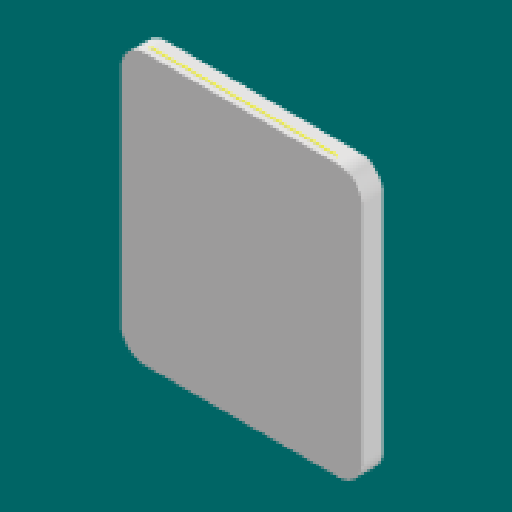
# Autodesk Inventor part: part1
Saved by Autodesk Inventor 2025.2 (Build 292293000, 293)
## iProperties
Created: 2025-05-26
Part Number: part1
Material: Generic
Document SubType Name: Modeling
Designer: ia088
Density: 1 g/cm^3
Appearance: Default
Author: ia088
Autodesk Inventor part; units mm, degrees
ref_plane "YZ Plane" through (0, 0, 0) normal (1, 0, 0) x (0, 1, 0)
ref_plane "XZ Plane" through (0, 0, 0) normal (0, 1, 0) x (-1, 0, 0)
ref_plane "XY Plane" through (0, 0, 0) normal (0, 0, 1) x (1, 0, 0)
ref_plane "Work Plane1" through (0, 0, 0) normal (0, 0, 1) x (1, 0, 0)
sketch "Sketch1" plane through (0, 0, 0) normal (0, 0, 1) x (1, 0, 0)
  line L0 (8.1543, -68.045) -> (8.1793, 2.155) projected
  line L1 (5.1793, 5.155) -> (-55.5957, 5.155) projected
  line L2 (-55.6207, -71.045) -> (5.1543, -71.045) projected
  line L3 (-58.5957, 2.155) -> (-58.6207, -68.045) projected
  arc A0 (8.1793, 2.155) -> (5.1793, 5.155) centre (5.1793, 2.155) ccw projected
  arc A1 (5.1543, -71.045) -> (8.1543, -68.045) centre (5.1543, -68.045) ccw projected
  arc A2 (-58.6207, -68.045) -> (-55.6207, -71.045) centre (-55.6207, -68.045) ccw projected
  arc A3 (-55.5957, 5.155) -> (-58.5957, 2.155) centre (-55.5957, 2.155) ccw projected
  circle A4 centre (-2.54, -13.97) radius 1.7875 projected
  circle A5 centre (-2.54, -13.97) radius 1.5875 projected
  circle A6 centre (-7.62, -66.04) radius 1.7875 projected
  circle A7 centre (-7.62, -66.04) radius 1.5875 projected
  circle A8 centre (-50.8, -15.24) radius 1.7875 projected
  circle A9 centre (-50.8, -15.24) radius 1.5875 projected
  circle A10 centre (-35.56, -66.04) radius 1.7875 projected
  circle A11 centre (-35.56, -66.04) radius 1.5875 projected
  line L4 (9.1793, 2.1536) -> (9.1543, -68.0464)
  arc A12 (5.1543, -72.045) -> (9.1543, -68.0464) centre (5.1543, -68.045) ccw
  line L5 (5.1543, -72.045) -> (-55.6207, -72.045)
  arc A13 (-59.6207, -68.0436) -> (-55.6207, -72.045) centre (-55.6207, -68.045) ccw
  line L6 (-59.6207, -68.0436) -> (-59.5957, 2.1564)
  arc A14 (-55.5957, 6.155) -> (-59.5957, 2.1564) centre (-55.5957, 2.155) ccw
  line L7 (-55.5957, 6.155) -> (5.1793, 6.155)
  arc A15 (9.1793, 2.1536) -> (5.1793, 6.155) centre (5.1793, 2.155) ccw
  point P0 (0, 0)
  dimension "d0" = 1
  constraints: 8 end point, 8 point on circle, 4 centre point, 7 other
  measures "d0" distance between parallel lines of L0 L4
extrude "Extrusion1" add sketch "Sketch1" along normal blind 2 contours A1 L2 A2 L3 A3 L1 A0 L0 | A4 | A5 | A6 | A7 | A8 | A9 | A10 | A11 | L4 A12 L5 A13 L6 A14 L7 A15
sketch "Sketch2" plane through (0, 0, 0) normal (0, 0, -1) x (-1, 0, 0)
  circle A0 centre (35.56, -66.04) radius 1.7875 projected
  circle A1 centre (7.62, -66.04) radius 1.5875 projected
  circle A2 centre (35.56, -66.04) radius 1.5875 projected
  circle A3 centre (50.8, -15.24) radius 1.5875 projected
  circle A4 centre (2.54, -13.97) radius 1.5875 projected
  circle A5 centre (50.8, -15.24) radius 1.4875
  circle A6 centre (2.54, -13.97) radius 1.4875
  circle A7 centre (35.56, -66.04) radius 1.4875
  circle A8 centre (7.62, -66.04) radius 1.4875
  point P0 (0, 0)
  dimension "d5" = 0.1
  dimension "d6" = 0.1
  dimension "d7" = 0.1
  dimension "d8" = 0.1
  constraints: 4 centre point
  measures "d5" radial gap between concentric circles of A3 A5
  measures "d6" radial gap between concentric circles of A4 A6
  measures "d7" radial gap between concentric circles of A2 A7
  measures "d8" radial gap between concentric circles of A1 A8
extrude "Extrusion2" add sketch "Sketch2" along normal blind 7 contours A5 | A6 | A7 | A8
fillet "Fillet1" radius 1 4 edges at (-1.0525, -13.97, 0) (-6.1325, -66.04, 0) (-34.0725, -66.04, 0) (-49.3125, -15.24, 0)
sketch "Sketch3" plane through (0, 0, 2) normal (0, 0, 1) x (1, 0, 0)
  line L0 (-59.5957, 2.1564) -> (-59.6207, -68.0436) projected
  arc A0 (-59.6207, -68.0436) -> (-55.6207, -72.045) centre (-55.6207, -68.045) ccw projected
  line L1 (-55.6207, -72.045) -> (5.1543, -72.045) projected
  arc A1 (5.1543, -72.045) -> (9.1543, -68.0464) centre (5.1543, -68.045) ccw projected
  line L2 (9.1543, -68.0464) -> (9.1793, 2.1536) projected
  arc A2 (9.1793, 2.1536) -> (5.1793, 6.155) centre (5.1793, 2.155) ccw projected
  line L3 (5.1793, 6.155) -> (-55.5957, 6.155) projected
  arc A3 (-55.5957, 6.155) -> (-59.5957, 2.1564) centre (-55.5957, 2.155) ccw projected
  line L4 (-55.5957, 7.655) -> (5.1793, 7.655)
  arc A4 (10.6793, 2.153) -> (5.1793, 7.655) centre (5.1793, 2.155) ccw
  line L5 (10.6793, 2.153) -> (10.6543, -68.047)
  arc A5 (5.1543, -73.545) -> (10.6543, -68.047) centre (5.1543, -68.045) ccw
  line L6 (5.1543, -73.545) -> (-55.6207, -73.545)
  arc A6 (-61.1207, -68.043) -> (-55.6207, -73.545) centre (-55.6207, -68.045) ccw
  line L7 (-61.1207, -68.043) -> (-61.0957, 2.157)
  arc A7 (-55.5957, 7.655) -> (-61.0957, 2.157) centre (-55.5957, 2.155) ccw
  point P0 (0, 0)
  dimension "d10" = 1.5
  constraints: 8 end point, 8 point on circle, 4 centre point, 7 other
  measures "d10" distance between parallel lines of L3 L4
ref_plane "Work Plane2" through (-53.34, -68.58, -4.65) normal (0, 0, -1) x (0, 1, 0)
extrude "Extrusion3" add sketch "Sketch3" against normal up to surface (6.65 mm away)
sketch "Sketch4" plane through (5.1543, -73.545, -4.65) normal (0, 0, -1) x (-1, 0, 0)
  arc A0 (-5.5, 5.498) -> (0, 0) centre (0, 5.5) ccw projected
  line L0 (60.775, 0) -> (0, 0) projected
  arc A1 (60.775, 0) -> (66.275, 5.502) centre (60.775, 5.5) ccw projected
  line L1 (66.25, 75.702) -> (66.275, 5.502) projected
  arc A2 (66.25, 75.702) -> (60.75, 81.2) centre (60.75, 75.7) ccw projected
  line L2 (-0.025, 81.2) -> (60.75, 81.2) projected
  arc A3 (-0.025, 81.2) -> (-5.525, 75.698) centre (-0.025, 75.7) ccw projected
  line L3 (-5.5, 5.498) -> (-5.525, 75.698) projected
  arc A4 (-0.025, 84.2) -> (-8.525, 75.697) centre (-0.025, 75.7) ccw
  line L4 (-0.025, 84.2) -> (60.75, 84.2)
  arc A5 (69.25, 75.703) -> (60.75, 84.2) centre (60.75, 75.7) ccw
  line L5 (69.25, 75.703) -> (69.275, 5.503)
  arc A6 (60.775, -3) -> (69.275, 5.503) centre (60.775, 5.5) ccw
  line L6 (60.775, -3) -> (0, -3)
  arc A7 (-8.5, 5.497) -> (0, -3) centre (0, 5.5) ccw
  line L7 (-8.5, 5.497) -> (-8.525, 75.697)
  point P0 (5.1543, 73.545)
  dimension "d13" = 3
  constraints: 8 end point, 8 point on circle, 4 centre point, 7 other
  measures "d13" distance between parallel lines of L3 L7
extrude "Extrusion4" add sketch "Sketch4" against normal up to surface (6.65 mm away)
sketch "Sketch5" plane through (0, 0, 2) normal (0, 0, 1) x (1, 0, 0)
  arc A0 (13.6793, 2.152) -> (5.1793, 10.655) centre (5.1793, 2.155) ccw projected
  line L0 (-55.5957, 10.655) -> (5.1793, 10.655) projected
  arc A1 (-55.5957, 10.655) -> (-64.0957, 2.158) centre (-55.5957, 2.155) ccw projected
  line L1 (-64.1207, -68.042) -> (-64.0957, 2.158) projected
  arc A2 (-64.1207, -68.042) -> (-55.6207, -76.545) centre (-55.6207, -68.045) ccw projected
  line L2 (5.1543, -76.545) -> (-55.6207, -76.545) projected
  arc A3 (5.1543, -76.545) -> (13.6543, -68.048) centre (5.1543, -68.045) ccw projected
  line L3 (13.6793, 2.152) -> (13.6543, -68.048) projected
  point P0 (0, 0)
extrude "Extrusion5" add sketch "Sketch5" along normal blind 1
sketch "Sketch6" plane through (5.1793, 10.655, -4.65) normal (0, 0, -1) x (-1, 0, 0)
  line L0 (-2.975, -78.7) -> (-3, -8.5) projected
  line L1 (63.775, -8.5) -> (63.8, -78.7) projected
  line L2 (-3, -8.5) -> (-8.475, -8.5)
  line L3 (-8.475, -8.5) -> (-8.475, -78.703)
  line L4 (-8.475, -78.703) -> (-3, -78.703)
  line L5 (-3, -78.703) -> (-3, -8.5)
  line L6 (-4.5302, -71.6525) -> (-6.9448, -71.6525)
  line L7 (-6.9448, -15.5504) -> (-4.5302, -15.5504)
  line L8 (-4.5302, -71.6525) -> (-6.9448, -15.5504) construction
  line L9 (-6.9448, -71.6525) -> (-4.5302, -15.5504) construction
  line L10 (-6.9448, -15.5504) -> (-4.5302, -15.5504)
  line L11 (-4.5302, -15.5504) -> (-4.5302, -35.5504)
  line L12 (-4.5302, -35.5504) -> (-6.9448, -35.5504)
  line L13 (-6.9448, -35.5504) -> (-6.9448, -15.5504)
  line L14 (-4.5302, -71.6525) -> (-6.9448, -71.6525)
  line L15 (-6.9448, -71.6525) -> (-6.9448, -51.6525)
  line L16 (-6.9448, -51.6525) -> (-4.5302, -51.6525)
  line L17 (-4.5302, -51.6525) -> (-4.5302, -71.6525)
  line L18 (-6.9448, -71.6525) -> (-6.9448, -51.6525)
  line L19 (-6.9448, -35.5504) -> (-6.9448, -15.5504)
  line L20 (-4.5302, -15.5504) -> (-4.5302, -35.5504)
  line L21 (-4.5302, -51.6525) -> (-4.5302, -71.6525)
  line L22 (60.775, -4.5) -> (0, -4.5) projected
  line L23 (0.025, -82.7) -> (60.8, -82.7) projected
  line L24 (30.3875, -4.5) -> (30.3875, -84.7093)
  line L25 (65.3052, -71.6525) -> (67.7198, -71.6525)
  line L26 (67.7198, -15.5504) -> (65.3052, -15.5504)
  line L27 (65.3052, -15.5504) -> (65.3052, -35.5504)
  line L28 (65.3052, -35.5504) -> (67.7198, -35.5504)
  line L29 (67.7198, -35.5504) -> (67.7198, -15.5504)
  line L30 (67.7198, -71.6525) -> (67.7198, -51.6525)
  line L31 (67.7198, -51.6525) -> (65.3052, -51.6525)
  line L32 (65.3052, -51.6525) -> (65.3052, -71.6525)
  line L33 (-8.5, -8.503) -> (-8.475, -78.703) projected
  arc A0 (-8.475, -78.703) -> (0.025, -87.2) centre (0.025, -78.7) ccw projected
  arc A1 (64.775, -8.4986) -> (60.775, -4.5) centre (60.775, -8.5) ccw projected
  line L34 (64.8, -78.6986) -> (64.775, -8.4986) projected
  arc A2 (60.8, -82.7) -> (64.8, -78.6986) centre (60.8, -78.7) ccw projected
  arc A3 (-3.975, -78.7014) -> (0.025, -82.7) centre (0.025, -78.7) ccw projected
  line L35 (-4, -8.5014) -> (-3.975, -78.7014) projected
  arc A4 (0, -4.5) -> (-4, -8.5014) centre (0, -8.5) ccw projected
  arc A5 (60.8, -81.7) -> (63.8, -78.7) centre (60.8, -78.7) ccw projected
  line L36 (60.8, -81.7) -> (0.025, -81.7) projected
  arc A6 (-2.975, -78.7) -> (0.025, -81.7) centre (0.025, -78.7) ccw projected
  line L37 (0, -5.5) -> (60.775, -5.5) projected
  arc A7 (63.775, -8.5) -> (60.775, -5.5) centre (60.775, -8.5) ccw projected
  arc A8 (0, -5.5) -> (-3, -8.5) centre (0, -8.5) ccw projected
  line L38 (60.8, -83.2) -> (0.025, -83.2)
  arc A9 (-4.475, -78.7016) -> (0.025, -83.2) centre (0.025, -78.7) ccw
  line L39 (-4.475, -78.7016) -> (-4.5, -8.5016)
  arc A10 (0, -4) -> (-4.5, -8.5016) centre (0, -8.5) ccw
  line L40 (0, -4) -> (60.775, -4)
  arc A11 (65.275, -8.4984) -> (60.775, -4) centre (60.775, -8.5) ccw
  line L41 (65.275, -8.4984) -> (65.3, -78.6984)
  arc A12 (60.8, -83.2) -> (65.3, -78.6984) centre (60.8, -78.7) ccw
  line L42 (67.7152, -78.6975) -> (67.6902, -8.4975)
  arc A13 (67.6902, -8.4975) -> (60.775, -1.5848) centre (60.775, -8.5) ccw
  line L43 (60.775, -1.5848) -> (0, -1.5848)
  arc A14 (0, -1.5848) -> (-6.9152, -8.5025) centre (0, -8.5) ccw
  line L44 (-6.9152, -8.5025) -> (-6.8902, -78.7025)
  arc A15 (-6.8902, -78.7025) -> (0.025, -85.6152) centre (0.025, -78.7) ccw
  line L45 (0.025, -85.6152) -> (60.8, -85.6152)
  arc A16 (60.8, -85.6152) -> (67.7152, -78.6975) centre (60.8, -78.7) ccw
  line L46 (63.8, -78.7) -> (69.5599, -78.7)
  line L47 (69.5599, -78.7) -> (-8.4749, -78.7429)
  line L48 (63.775, -8.5) -> (69.275, -8.497)
  line L49 (69.275, -8.497) -> (-8.5, -8.5037)
  line L50 (60.8, -81.7) -> (60.8, -87.2)
  line L51 (60.8, -87.2) -> (60.775, 0)
  line L52 (0, -5.5) -> (0, 0)
  line L53 (0, 0) -> (0.025, -87.2)
  point P0 (5.1793, -10.655)
  point P1 (-5.7375, -43.6014)
  point P2 (-4.5302, -15.5504)
  point P3 (60.7755, -1.5848)
  point P4 (60.7761, -4)
  point P5 (65.275, -8.4973)
  point P6 (67.6902, -8.4971)
  point P7 (0, -4)
  point P8 (0, -1.5848)
  point P9 (-6.9152, -8.5)
  point P10 (-4.5, -8.5)
  point P11 (0.0245, -85.6152)
  point P12 (0.0239, -83.2)
  point P13 (-4.4748, -78.7407)
  point P14 (-6.8901, -78.7421)
  point P15 (60.8, -83.2)
  point P16 (60.8, -85.6152)
  point P17 (67.7152, -78.701)
  point P18 (65.3, -78.7023)
  dimension "d0" = 1
  dimension "d18" = 20
  dimension "d19" = 20
  dimension "d22" = 0.5
  constraints: 90 end point, 17 point on circle, 12 parallel, 10 symmetric about line, 8 centre point, 7 perpendicular, 5 horizontal, 3 midpoint, 1 point on line, 14 other
  measures "d18" distance of L10.end L11.end
  measures "d19" distance of L14.end L15.end
  measures "d22" distance between parallel lines of L23 L38
extrude "Extrusion6" cut sketch "Sketch6" against normal blind 5.65 contours A9 L53 A15 L47 | L2 A14 L52 A10 | L51 A13 L48 A11 | L44 L12 L13 L7 | L7 L11 L12 L44 | L44 L16 L17 L6 | L6 L15 L16 L44 | A12 L47 A16 L50 | L42 L28 L27 L26 | L26 L29 L28 L42 | L42 L31 L30 L25 | L25 L32 L31 L42
body "Solid1"
